LatchMechRetainerConcept v1 (Autodesk Fusion 360 design; units mm, degrees)
Autodesk Fusion 360 part; units mm, degrees
sketch "Sketch1" plane through (0, 0, 0) normal (0, 1, 0) x (1, 0, 0)
  circle A0 centre (0, 0) radius 25
  circle A1 centre (0, 0) radius 45
  dimension "d1" = 50
  dimension "d2" = 20
  constraint coincident A0.centre A1.centre
  measures "d1" diameter of A0
extrude "Extrude1" add sketch "Sketch1" along normal blind 5 makes body 1
sketch "Sketch2" plane through (0, 5, 0) normal (0, 1, 0) x (-1, 0, 0)
  circle A0 centre (0, 0) radius 25
  circle A1 centre (0, 0) radius 45
  line L0 (0, 0) -> (28.7013, -69.291)
  line L1 (28.7013, -69.291) -> (-28.7013, -69.291) construction
  line L2 (-28.7013, -69.291) -> (0, 0)
  circle A2 centre (0, 0) radius 75
  dimension "d5" = 45
  dimension "d6" = 150
  constraint coincident A0.centre A1.centre
  constraint equal L0 L2
  constraint coincident L0.end A2
  constraint horizontal L1
  measures "d5" angle of L0 L2
  measures "d6" diameter of A2
extrude "Extrude2" add sketch "Sketch2" against normal blind 150 contours A1 L0 L2 A2 picked at (21.7778, -61.1033) bodies 1
pattern_circular "C-Pattern1" count 3 over 360 about axis through (0, 0, 0) along (0, 1, 0) of "Extrude2"
sketch "Sketch3" plane through (0, -145, 0) normal (0, -1, 0) x (1, 0, 0)
  arc A0 (-28.7013, -69.291) -> (28.7013, -69.291) centre (0, 0) ccw
  line L0 (28.7013, -69.291) -> (17.2208, -41.5746)
  arc A1 (-17.2208, -41.5746) -> (17.2208, -41.5746) centre (0, 0) ccw
  line L1 (-17.2208, -41.5746) -> (-28.7013, -69.291)
  circle A2 centre (0, 0) radius 45
  circle A3 centre (0, 0) radius 50
  dimension "d11" = 5
  constraint coincident A0.centre A1.centre
  constraint coincident L0.end A2
extrude "Extrude3" add sketch "Sketch3" along normal blind 15 contours L0 L1 A2 A3 | L0 A1 L1 A2 A3 bodies 1
ref_plane "WorkPlane1" through (0, -175, 0) normal (0, -1, 0) x (1, 0, 0)
sketch "Sketch4" plane through (0, -175, 0) normal (0, -1, 0) x (1, 0, 0)
  circle A0 centre (0, 0) radius 20
  circle A1 centre (0, 0) radius 52.5
  dimension "d15" = 40
  dimension "d16" = 105
  constraint coincident A0.centre A1.centre
  constraint concentric A0 A1
  measures "d15" diameter of A0
  measures "d16" diameter of A1
extrude "Extrude4" add sketch "Sketch4" along normal blind 5 separate body makes body 2
sketch "Sketch5" plane through (0, -175, 0) normal (0, 1, 0) x (-1, 0, 0)
  circle A0 centre (0, 0) radius 20
  circle A1 centre (0, 0) radius 52.5
  circle A2 centre (0, 0) radius 50
  arc A3 (19.1342, -46.194) -> (49.5722, 6.5263) centre (0, 0) ccw
  arc A4 (-19.1342, -46.194) -> (19.1342, -46.194) centre (0, 0) ccw
  arc A5 (-49.5722, 6.5263) -> (-19.1342, -46.194) centre (0, 0) ccw
  arc A6 (-30.4381, 39.6677) -> (-49.5722, 6.5263) centre (0, 0) ccw
  arc A7 (30.4381, 39.6677) -> (-30.4381, 39.6677) centre (0, 0) ccw
  arc A8 (49.5722, 6.5263) -> (30.4381, 39.6677) centre (0, 0) ccw
extrude "Extrude5" add sketch "Sketch5" along normal blind 29 separate body contours A1 makes body 3
combine "Combine1" operation add target body 3 tool bodies 2
copy_body "Body->Comp1" bodies 1 removing the originals makes body 4 in component "Component"
copy_body "Body->Comp2" bodies 3 removing the originals makes body 5 in component "Component'"
sketch "Sketch6" plane through (0, 0, 0) normal (0, -1, 0) x (1, 0, 0)
  circle A0 centre (0, 0) radius 25
  arc A1 (-44.615, 5.8737) -> (-17.2208, -41.5746) centre (0, 0) ccw
  arc A2 (-17.2208, -41.5746) -> (17.2208, -41.5746) centre (0, 0) ccw
  arc A3 (17.2208, -41.5746) -> (44.615, 5.8737) centre (0, 0) ccw
  arc A4 (44.615, 5.8737) -> (27.3943, 35.7009) centre (0, 0) ccw
  arc A5 (27.3943, 35.7009) -> (-27.3943, 35.7009) centre (0, 0) ccw
  arc A6 (-27.3943, 35.7009) -> (-44.615, 5.8737) centre (0, 0) ccw
  circle A7 centre (0, 0) radius 42.5
  line L0 (0, 0) -> (27.3943, 35.7009)
  line L1 (0, 0) -> (44.615, 5.8737)
  dimension "d25" = 85
  constraint coincident A0.centre A1.centre
  constraint coincident A4.end A5.start
  constraint coincident A3.end A4.start
  measures "d25" diameter of A7
extrude "Extrude1'" add sketch "Sketch6" along normal blind 100 contours A4 A7 L0 L1 bodies 4 in component "Component"
pattern_circular "C-Pattern1'" count 3 over 360 about axis through (0, -145, 0) along (0, -1, 0) of "Extrude1'" in component "Component"
move_face "OffsetFaces1" offset 5 1 faces at (-24.8758, 1.6667, 2.4892) on bodies 4 in component "Component"
move_face "OffsetFaces2" offset 15 1 faces at (0, 5, -52.7164) on bodies 4 in component "Component"
component "Component" placed x (1, 0, 0) y (0, 1, 0) z (0, 0, 1) at (0, 0, 0)
component "Component'" placed x (1, 0, 0) y (0, 1, 0) z (0, 0, 1) at (0, -39.0946, 0)
